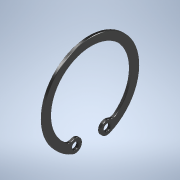
# Autodesk Inventor part: Seger
Saved by Autodesk Inventor 2020.2 (Build 242310000, 310)
## iProperties
Created: 2020-07-09
Part Number: Seger
Material: Ogólny
Document SubType Name: Modeling
Designer: Artur Lenart
Density: 1 g/cm^3
Appearance: Stal nierdzewna — jasna
Author: Artur Lenart
Autodesk Inventor part; units mm, degrees
ref_plane "YZ Plane" through (0, 0, 0) normal (1, 0, 0) x (0, 1, 0)
ref_plane "XZ Plane" through (0, 0, 0) normal (0, 1, 0) x (-1, 0, 0)
ref_plane "XY Plane" through (0, 0, 0) normal (0, 0, 1) x (1, 0, 0)
sketch "Szkic1" plane through (0, 0, 0) normal (1, 0, 0) x (0, 1, 0)
  arc A0 (-8.3149, -3.4442) -> (-8.3149, 3.4442) centre (0, 0) ccw
  arc A1 (-6.9291, -2.8701) -> (-6.694, -3.3823) centre (0, 0) ccw construction
  line L0 (0, 0) -> (-6.5826, 2.7266)
  line L1 (0, 0) -> (-6.5826, -2.7266)
  line L2 (-11.9129, 0) -> (12.4855, 0) projected
  circle A2 centre (-7.1601, 2.9658) radius 0.625
  line L3 (-6.9291, 2.8701) -> (-7.1601, 2.9658) construction
  arc A3 (-8.3149, 3.4442) -> (-6.0415, 3.5238) centre (-7.1601, 2.9658) ccw
  circle A4 centre (-7.1601, -2.9658) radius 0.625
  arc A5 (-6.3801, -3.9426) -> (-6.0415, -3.5238) centre (-7.1601, -2.9658) ccw construction
  arc A6 (-6.694, -3.3823) -> (-6.3801, -3.9426) centre (0, 0) ccw construction
  arc A7 (-6.3801, -3.9426) -> (-5.9385, -4.5809) centre (0, 0) ccw construction
  arc A8 (-6.694, 3.3823) -> (-6.9291, 2.8701) centre (0, 0) ccw construction
  line L4 (-6.5826, 2.7266) -> (-8.3149, 3.4442) construction
  line L5 (-6.5826, -2.7266) -> (-8.3149, -3.4442) construction
  arc A9 (-6.3801, 3.9426) -> (-6.694, 3.3823) centre (0, 0) ccw construction
  arc A10 (-5.9385, 4.5809) -> (-6.0415, 3.5238) centre (-5.1467, 3.9701) ccw
  arc A11 (-6.0415, -3.5238) -> (-5.9385, -4.5809) centre (-5.1467, -3.9701) ccw
  arc A12 (-5.9385, 4.5809) -> (-6.3801, 3.9426) centre (0, 0) ccw construction
  arc A13 (-6.0415, 3.5238) -> (-6.3801, 3.9426) centre (-7.1601, 2.9658) ccw construction
  arc A14 (-6.0415, -3.5238) -> (-8.3149, -3.4442) centre (-7.1601, -2.9658) ccw
  arc A15 (-5.9385, -4.5809) -> (-5.9385, 4.5809) centre (0, 0) ccw
  dimension "d0" = 18
  dimension "d1" = 15
  dimension "d2" = 45
  dimension "d3" = 1.25
  dimension "d4" = 0.25
  dimension "d5" = 2
  constraints: 32 point on circle, 16 centre point, 10 end point, 6 point on line, 5 symmetric about line, 4 coincident, 2 tangent, 4 other
  measures "d0" diameter of A0
  measures "d1" diameter of A1
  measures "d2" angle of L1 L0
  measures "d3" diameter of A2
  measures "d4" distance of L3.start L3.end
  measures "d5" diameter of A10
extrude "Wyciągnięcie proste1" add sketch "Szkic1" along normal blind 0.5 contours A14 A11 A15 L2 A0 | L2 A15 A10 A3 A0
chamfer "Faza1" distance 0.05 angle 45 16 edges at (0.5, 7.5, 0) (0.5, -6.1419, -4.0672) (0.5, -7.1163, -1.7166) (0.5, 9, 0) (0.5, -7.1163, 1.7166) (0.5, -6.1419, 4.0672) (0, 7.5, 0) (0, -6.1419, -4.0672) (0, -7.1163, -1.7166) (0, 9, 0) (0, -7.1163, 1.7166) (0, -6.1419, 4.0672) (0, -7.7851, 2.9658) (0.5, -7.7851, 2.9658) (0, -7.7851, -2.9658) (0.5, -7.7851, -2.9658)
